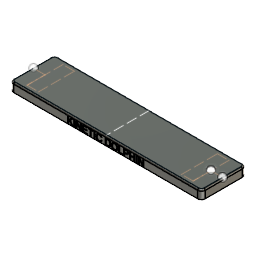
Kinetic Dolphin (Autodesk Fusion 360 archive; units mm, degrees)
design "Frame_Base"
part number: 2026-05-20-12-45-40-132
Autodesk Fusion 360 part; units mm, degrees
sketch "Sketch_01_Sketch_Base_Profile" plane through (0, 0, 0) normal (0, 0, 1) x (1, 0, 0)
  line L0 (6, 0) -> (294, 0)
  line L1 (300, 6) -> (300, 64)
  line L2 (294, 70) -> (6, 70)
  line L3 (0, 64) -> (0, 6)
  arc A0 (6, 70) -> (0, 64) centre (6, 64) ccw
  arc A1 (0, 6) -> (6, 0) centre (6, 6) ccw
  arc A2 (300, 64) -> (294, 70) centre (294, 64) ccw
  arc A3 (294, 0) -> (300, 6) centre (294, 6) ccw
  point P0 (300, 0)
  point P1 (0, 70)
  dimension "d1" = 300
  dimension "d2" = 70
  dimension "d3" = 6
  constraint horizontal L0
  constraint vertical L1
  constraint horizontal L2
  constraint vertical L3
  constraint coincident P1 L2
  constraint coincident P1 L3
  constraint tangent L2 A0
  constraint tangent L3 A0
  constraint coincident origin L0
  constraint coincident origin L3
  constraint tangent L0 A1
  constraint tangent L3 A1
  constraint equal A0 A1
  constraint tangent L1 A2
  constraint tangent L2 A2
  constraint equal A0 A2
  constraint coincident P0 L0
  constraint coincident P0 L1
  constraint tangent L0 A3
  constraint tangent L1 A3
  constraint equal A0 A3
  measures "d1" distance of origin P0
  measures "d2" distance of origin P1
  measures "d3" radius of A0
extrude "Extrude_Base_14mm" add sketch "Sketch_01_Sketch_Base_Profile" along normal blind 14
fillet "Fillet_Base_Top_Edges_2mm" radius 2 8 edges at (150, 0, 14) (298.2426, 1.7574, 14) (300, 35, 14) (298.2426, 68.2426, 14) (150, 70, 14) (1.7574, 68.2426, 14) (0, 35, 14) (1.7574, 1.7574, 14)
fillet "Fillet_Base_Bottom_Edges_0_5mm" radius 0.5 8 edges at (300, 35, 0) (298.2426, 68.2426, 0) (150, 70, 0) (1.7574, 68.2426, 0) (0, 35, 0) (1.7574, 1.7574, 0) (150, 0, 0) (298.2426, 1.7574, 0)
sketch "Sketch_02_Sketch_Column_Footprints" plane through (0, 0, 14) normal (0, 0, 1) x (-1, 0, 0)
  line L0 (-6, -2) -> (-294, -2)
  arc A0 (-294, -2) -> (-298, -6) centre (-294, -6) ccw
  line L1 (-298, -6) -> (-298, -64)
  arc A1 (-298, -64) -> (-294, -68) centre (-294, -64) ccw
  line L2 (-294, -68) -> (-6, -68)
  arc A2 (-6, -68) -> (-2, -64) centre (-6, -64) ccw
  line L3 (-2, -64) -> (-2, -6)
  arc A3 (-2, -6) -> (-6, -2) centre (-6, -6) ccw
  line L4 (-20.0245, -35) -> (-2.0245, -35) construction
  line L5 (-150, -68) -> (-150, -2) construction
  line L6 (-279.9755, -35) -> (-297.9755, -35) construction
  line L7 (-20.0245, -35) -> (-20.0245, -7) construction
  line L8 (-20.0245, -7) -> (-38.0245, -7) construction
  line L9 (-38.0245, -7) -> (-38.0245, -63) construction
  line L10 (-38.0245, -63) -> (-20.0245, -63) construction
  line L11 (-20.0245, -63) -> (-20.0245, -7) construction
  line L12 (-261.9755, -7) -> (-261.9755, -63) construction
  line L13 (-279.9755, -35) -> (-279.9755, -7) construction
  line L14 (-279.9755, -7) -> (-261.9755, -7) construction
  line L15 (-261.9755, -63) -> (-279.9755, -63) construction
  line L16 (-279.9755, -63) -> (-279.9755, -7) construction
  dimension "d11" = 18
  dimension "d12" = 28
  dimension "d13" = 18
  dimension "d14" = 56
  constraint perpendicular L3 L4
  constraint midpoint L2 L5.start
  constraint midpoint L0 L5.end
  constraint symmetric L4.start L5 L6.start
  constraint symmetric L4.end L5 L6.end
  constraint perpendicular L4 L7
  constraint horizontal L8
  constraint vertical L9
  constraint horizontal L10
  constraint vertical L11
  constraint symmetric L5 L7.end L13.end
  constraint symmetric L5 L8.end L12.start
  constraint symmetric L5 L9.end L12.end
  constraint symmetric L5 L10.end L15.end
  measures "d11" distance of L4.start L4.end
  measures "d12" distance of L4.start L7.end
  measures "d13" distance of L7.end L8.end
  measures "d14" distance of L7.end L10.end
sketch "Sketch_03_Front_Text" plane through (0, 0, 0) normal (0, -1, 0) x (1, 0, 0)
  line L0 (6, 0.5) -> (294, 0.5)
  line L1 (294, 0.5) -> (294, 12)
  line L2 (294, 12) -> (6, 12)
  line L3 (6, 12) -> (6, 0.5)
  line L4 (6, 0.5) -> (294, 0.5) construction
  line L5 (294, 0.5) -> (294, 12) construction
  line L6 (294, 12) -> (6, 12) construction
  line L7 (6, 12) -> (6, 0.5) construction
  dimension "d15" = 10
  text T0 "KINETIC DOLPHIN" font "Arial" height 10 align centre middle in box 288 x 11.5 at (6, 0.5) x (1, 0) y (0, 1) spacing 1 kerned
  constraint coincident L1.end
  constraint coincident L0.start
extrude "Cut_Front_Text_1mm" cut sketch "Sketch_03_Front_Text" against normal blind 1 text T0
equation "d16 = 'KINETIC DOLPHIN'"
named bodies: "Frame_Base_Body"
